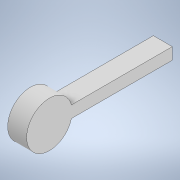
# Autodesk Inventor part: Pata1_v1
Saved by Autodesk Inventor 2021 (Build 250183000, 183)
## iProperties
Created: 2021-06-19
Part Number: Pata1_v1
Material: Genérico
Document SubType Name: Modeling
Designer: Juan
Density: 1 g/cm^3
Appearance: Valor por defecto
Author: Juan
Autodesk Inventor part; units mm, degrees
ref_plane "YZ Plane" through (0, 0, 0) normal (1, 0, 0) x (0, 1, 0)
ref_plane "XZ Plane" through (0, 0, 0) normal (0, 1, 0) x (-1, 0, 0)
ref_plane "XY Plane" through (0, 0, 0) normal (0, 0, 1) x (1, 0, 0)
sketch "Boceto1" plane through (0, 0, 0) normal (0, 0, 1) x (1, 0, 0)
  point P0 (0, 0)
sketch "Boceto2" plane through (0, 0, 0) normal (1, 0, 0) x (0, 1, 0)
  circle A0 centre (0, 0) radius 48
  dimension "d0" = 96
  constraints: 1 centre point, 1 coincident
  measures "d0" diameter of A0
extrude "Extrusión1" add sketch "Boceto2" along normal blind 40
sketch "Boceto3" plane through (40, 0, 0) normal (1, 0, 0) x (0, 0, -1)
  circle A0 centre (0, 0) radius 48 projected
  arc A1 (48, 0) -> (46.3644, 12.4233) centre (0, 0) ccw
  arc A2 (46.3644, -12.4233) -> (48, 0) centre (0, 0) ccw
  line L0 (46.3644, -12.4233) -> (212.8644, -12.4233)
  line L1 (46.3644, 12.4233) -> (212.8644, 12.4233)
  line L2 (211.2289, 0) -> (259.2289, 0)
  line L3 (259.2289, 0) -> (259.2289, 12.4233)
  line L4 (259.2289, 0) -> (259.2289, -12.4233)
  line L5 (259.2289, -12.4233) -> (212.8644, -12.4233)
  line L6 (259.2289, 12.4233) -> (212.8644, 12.4233)
  constraints: 14 end point, 7 point on circle, 3 horizontal, 2 centre point, 2 perpendicular, 1 coincident, 1 parallel, 1 vertical
extrude "Extrusión2" add sketch "Boceto3" against normal blind 40 contours A0 L1 L6 L3 L4 L5 L0
